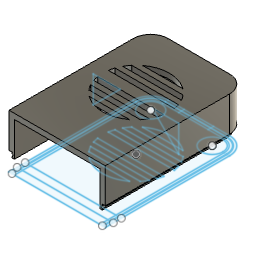
USB2CAN module enclosure v9 (Autodesk Fusion 360 design; units mm, degrees)
Autodesk Fusion 360 part; units mm, degrees
note: some values were not read from the file. Chosen so that the rebuilt part matches the saved one: which bodies a step acts on; which face or edge a step refers to.
sketch "PCB" plane through (0, 0, 0) normal (0, 0, 1) x (1, 0, 0)
  line L0 (-15.5, -25) -> (15.5, -25)
  line L1 (15.5, -25) -> (15.5, 21)
  line L2 (11.5, 25) -> (-11.5, 25)
  line L3 (-15.5, 21) -> (-15.5, -25)
  arc A0 (-11.5, 25) -> (-15.5, 21) centre (-11.5, 21) ccw
  arc A1 (15.5, 21) -> (11.5, 25) centre (11.5, 21) ccw
  circle A2 centre (-11.5, 21) radius 1.5
  circle A3 centre (11.5, 21) radius 1.5
  line L4 (-15.5, -24) -> (15.5, -24)
  circle A4 centre (0, 9) radius 1.75
  circle A5 centre (0, 9) radius 5
  dimension "d3" = 4
  dimension "d4" = 3
  dimension "d5" = 3
  dimension "d6" = -1
  dimension "d55" = 3.5
  dimension "d58" = 10
  constraint horizontal L0
  constraint perpendicular L0 L1
  constraint parallel L0 L2
  constraint parallel L1 L3
  constraint tangent L2 A0
  constraint tangent L3 A0
  constraint tangent L2 A1
  constraint tangent L1 A1
  constraint equal A0 A1
  constraint concentric A0 A2
  constraint concentric A1 A3
  constraint concentric A4 A5
  measures "d3" radius of A0
  measures "d4" diameter of A2
  measures "d5" diameter of A3
  measures "d55" diameter of A4
  measures "d58" diameter of A5
sketch "Base" plane through (0, 0, 0) normal (0, 0, 1) x (1, 0, 0)
  line L0 (11.5, 25.5) -> (-11.5, 25.5)
  arc A0 (-11.5, 25.5) -> (-16, 21) centre (-11.5, 21) ccw
  line L1 (-16, 21) -> (-16, -25.5)
  line L2 (-18, -25.5) -> (18, -25.5)
  line L3 (16, -25.5) -> (16, 21)
  arc A1 (16, 21) -> (11.5, 25.5) centre (11.5, 21) ccw
  line L4 (11.5, 27.5) -> (-11.5, 27.5)
  arc A2 (-11.5, 27.5) -> (-18, 21) centre (-11.5, 21) ccw
  line L5 (-18, 21) -> (-18, -25.5)
  line L6 (18, -25.5) -> (18, 21)
  arc A3 (18, 21) -> (11.5, 27.5) centre (11.5, 21) ccw
  line L7 (5.5, 25.5) -> (5.5, 27.5)
  line L8 (-5.5, 25.5) -> (-5.5, 27.5)
  line L9 (17.1, -25.5) -> (17.1, 21)
  arc A4 (17.1, 21) -> (11.5, 26.6) centre (11.5, 21) ccw
  line L10 (11.5, 26.6) -> (-11.5, 26.6)
  arc A5 (-11.5, 26.6) -> (-17.1, 21) centre (-11.5, 21) ccw
  line L11 (-17.1, 21) -> (-17.1, -25.5)
  line L12 (16.9, -25.5) -> (16.9, 21)
  arc A6 (16.9, 21) -> (11.5, 26.4) centre (11.5, 21) ccw
  line L13 (11.5, 26.4) -> (-11.5, 26.4)
  arc A7 (-11.5, 26.4) -> (-16.9, 21) centre (-11.5, 21) ccw
  line L14 (-16.9, 21) -> (-16.9, -25.5)
  dimension "d40" = 0.9
  constraint tangent A0 L1
  constraint tangent L0 A0
  constraint tangent L3 A1
  constraint tangent L0 A1
  constraint tangent L4 A2
  constraint tangent L6 A3
  constraint tangent A2 L5
  constraint tangent L4 A3
  constraint coincident L1.end L2
  constraint coincident L3.start L2
  constraint coincident L0 L8.start
  constraint coincident L0 L7.start
  constraint coincident L4 L7.end
  constraint coincident L4 L8.end
  constraint concentric A3 A4
  constraint concentric A2 A5
  constraint tangent A5 L11
  constraint tangent L10 A5
  constraint tangent A4 L10
  constraint tangent L9 A4
  constraint coincident L2 L11.end
  constraint coincident L2 L9.start
sketch "Supports" plane through (0, 0, 0) normal (0, 0, 1) x (1, 0, 0)
  line L0 (-16, -24) -> (16, -24)
  circle A0 centre (-11.5, 21) radius 1.25
  circle A1 centre (-11.5, 21) radius 2.5
  line L1 (-16, -25) -> (16, -25)
  circle A2 centre (11.5, 21) radius 2.5
  circle A3 centre (11.5, 21) radius 1.25
  line L2 (-16, -24) -> (-16, -25)
  line L3 (16, -24) -> (16, -25)
  dimension "d17" = 2.5
  dimension "d18" = 2.5
  dimension "d20" = 5
  dimension "d21" = 5
  dimension "d22" = 1
  constraint horizontal L1
  constraint perpendicular L1 L2
  constraint perpendicular L1 L3
  measures "d17" diameter of A0
  measures "d18" diameter of A3
  measures "d20" diameter of A1
  measures "d21" diameter of A2
  measures "d22" distance of L0 L1
extrude "Extrude1" add sketch "Base" along normal blind 1 contours L0 A0 L1 L2 L3 A1 makes body 1
extrude "Extrude2" add sketch "Base" along normal blind 5 contours L0 L2 L3 A1 L7 L12 A6 L13 | L0 A0 L1 L2 L8 L13 A7 L14 | L2 L7 L9 A4 L10 L12 A6 L13 | L2 L8 L10 A5 L11 L13 A7 L14 | L2 L4 L6 A3 L7 L9 A4 L10 | L2 L4 A2 L5 L8 L10 A5 L11 bodies 1
extrude "Extrude3" add sketch "Base" along normal blind 2 contours L0 L7 L8 L13 | L7 L8 L10 L13 | L4 L7 L8 L10 bodies 1
extrude "Extrude4" add sketch "Supports" along normal blind 3 bodies 1
extrude "Extrude5" cut sketch "Supports" along normal blind 5 contours A0 | A3 bodies 1
extrude "Extrude6" add sketch "Base" along normal blind 3 contours L0 L7 L8 L13 | L7 L8 L10 L13 | L4 L7 L8 L10 bodies 1
extrude "Extrude7" add sketch "Base" along normal blind 2 from surface at 5 contours L2 L4 L6 A3 L7 L9 A4 L10 | L2 L4 A2 L5 L8 L10 A5 L11 bodies 1
extrude "Extrude8" add sketch "Supports" along normal blind 5 contours A0 | A3 bodies 1
pipe "Pipe2" add diameter 0.75 path "Base" along L11 A5 L10 A4 L9 separate body makes body 2
move_body "Move2" bodies 2 to x (1, 0, 0) y (0, 1, 0) z (0, 0, 1) at (0, 0, 6)
split "Split1" by plane through (-5.5, 25.5, 0) normal (1, 0, 0) bodies 2 makes body 3 at (17.1151, -10, 5.6253)
split "Split2" by plane through (5.5, 25.5, 0) normal (-1, 0, 0) bodies 3 makes body 4 at (1.8333, 26.8481, 5.7188)
delete_body "RemoveBody1" bodies 4
combine "Combine1" operation add target body 1 tool bodies 2 3
extrude "Extrude9" cut sketch "PCB" along normal blind 2 contours A4 bodies 1
extrude "Extrude10" add sketch "PCB" against normal blind 1.5 contours L0 L1 L3 L4 | A2 | A3 | A5 bodies 1
sketch "Sketch4" plane through (0, 0, 0) normal (0, 0, 1) x (1, 0, 0)
  line L0 (11.5, 25.5) -> (-11.5, 25.5)
  line L1 (-16, 21) -> (-16, -25.5)
  line L2 (11.5, 27.5) -> (-11.5, 27.5)
  line L3 (11.5, 26.4) -> (-11.5, 26.4)
  line L4 (-5.5, 25.5) -> (-5.5, 27.5)
  line L5 (18, -25.5) -> (18, 21)
  arc A0 (18, 21) -> (11.5, 27.5) centre (11.5, 21) ccw
  arc A1 (16.9, 21) -> (11.5, 26.4) centre (11.5, 21) ccw
  line L6 (5.5, 25.5) -> (5.5, 27.5)
  arc A2 (-11.5, 25.5) -> (-16, 21) centre (-11.5, 21) ccw
  arc A3 (-11.5, 27.5) -> (-18, 21) centre (-11.5, 21) ccw
  line L7 (-18, 21) -> (-18, -25.5)
  arc A4 (-11.5, 26.6) -> (-17.1, 21) centre (-11.5, 21) ccw
  line L8 (17.1, -25.5) -> (17.1, 21)
  arc A5 (-11.5, 26.4) -> (-16.9, 21) centre (-11.5, 21) ccw
  line L9 (16, -25.5) -> (16, 21)
  line L10 (16.9, -25.5) -> (16.9, 21)
  line L11 (-17.1, 21) -> (-17.1, -25.5)
  arc A6 (17.1, 21) -> (11.5, 26.6) centre (11.5, 21) ccw
  line L12 (-16.9, 21) -> (-16.9, -25.5)
  line L13 (11.5, 26.6) -> (-11.5, 26.6)
  arc A7 (16, 21) -> (11.5, 25.5) centre (11.5, 21) ccw
  line L14 (-18, -25.5) -> (18, -25.5)
  circle A8 centre (-11.5, 21) radius 4
  circle A9 centre (11.5, 21) radius 4
  line L15 (12.339, 6) -> (-12.339, 6)
  line L16 (12.339, 2) -> (-12.339, 2)
  line L17 (11.8427, 0) -> (-11.8427, 0)
  line L18 (10.9659, -2) -> (-10.9659, -2)
  line L19 (9.6047, -4) -> (-9.6047, -4)
  line L20 (7.5, -6) -> (-7.5, -6)
  line L21 (11.8427, 8) -> (-11.8427, 8)
  line L22 (10.9659, 10) -> (-10.9659, 10)
  line L23 (9.6047, 12) -> (-9.6047, 12)
  line L24 (7.5, 14) -> (-7.5, 14)
  arc A10 (-7.5, -6) -> (7.5, -6) centre (0, 4) ccw
  arc A11 (7.5, 14) -> (-7.5, 14) centre (0, 4) ccw
  arc A12 (-9.6047, 12) -> (-10.9659, 10) centre (0, 4) ccw
  arc A13 (10.9659, 10) -> (9.6047, 12) centre (0, 4) ccw
  arc A14 (-11.8427, 8) -> (-12.339, 6) centre (0, 4) ccw
  arc A15 (12.339, 6) -> (11.8427, 8) centre (0, 4) ccw
  arc A16 (-12.339, 2) -> (-11.8427, 0) centre (0, 4) ccw
  arc A17 (-10.9659, -2) -> (-9.6047, -4) centre (0, 4) ccw
  arc A18 (9.6047, -4) -> (10.9659, -2) centre (0, 4) ccw
  arc A19 (11.8427, 0) -> (12.339, 2) centre (0, 4) ccw
  line L25 (-18, -22.5) -> (18, -22.5)
  line L26 (-18, -19.5) -> (18, -19.5)
  line L27 (-16, 4, 8) -> (-16, 4, 18)
  line L28 (16, 4, 8) -> (16, 4, 18)
  line L29 (-16, 4, 8) -> (-6, 4, 18)
  line L30 (6, 4, 18) -> (16, 4, 8)
  line L31 (-16, 4, 18) -> (-6, 4, 18)
  line L32 (6, 4, 18) -> (16, 4, 18)
  point P0 (0, 4)
  point P1 (0, 4)
  point P2 (0, 4)
  dimension "d61" = 0.9
  dimension "d62" = 0.9
  dimension "d63" = 0.9
  dimension "d64" = 0.9
  dimension "d65" = 8
  dimension "d66" = 8
  dimension "d69" = 25
  dimension "d96" = -3
  dimension "d97" = -6
  dimension "d103" = 10
  dimension "d104" = 10
  dimension "d105" = 10
  dimension "d106" = 10
  constraint coincident P2 P1
  constraint tangent L1 A2
  constraint tangent L0 A2
  constraint tangent L9 A7
  constraint tangent L0 A7
  constraint tangent L2 A3
  constraint tangent L5 A0
  constraint tangent A3 L7
  constraint tangent L2 A0
  constraint coincident L1.end L14
  constraint coincident L9.start L14
  constraint coincident L4.start L0
  constraint coincident L6.start L0
  constraint coincident L6.end L2
  constraint coincident L4.end L2
  constraint concentric A0 A6
  constraint concentric A3 A4
  constraint tangent A4 L11
  constraint tangent A4 L13
  constraint tangent A6 L13
  constraint tangent L8 A6
  constraint coincident L11.end L14
  constraint coincident L8.start L14
  constraint concentric A2 A8
  constraint concentric A0 A9
  constraint parallel L15 L21
  constraint concentric A10 A18
  constraint coincident L24.start A18
  constraint coincident L24.end A18
  constraint concentric A11 A18
  constraint concentric A11 A12
  constraint concentric A12 A14
  constraint concentric A13 A18
  constraint coincident L15.start A18
  constraint concentric A14 A16
  constraint concentric A15 A18
  constraint coincident L17.start A18
  constraint coincident L18.end A16
  constraint concentric A16 A17
  constraint concentric A18 A19
  measures "d62" distance of L5 L8
  measures "d63" distance of L2 L13
  measures "d64" distance of L7 L11
  measures "d65" diameter of A8
  measures "d66" diameter of A9
  measures "d69" diameter of A18
extrude "Extrude12" add sketch "Sketch4" against normal blind 1 from surface at 19 separate body contours L0 L1 A2 L9 A7 L26 | L0 L3 A1 L6 L9 L10 A7 L26 | L0 L3 L4 L6 | L0 L1 L3 L4 A2 A5 L12 L26 | L3 A1 L6 L8 L10 A6 L13 L26 | L3 L4 L6 L13 | L9 L10 L25 L26 | L1 L9 L25 L26 | L3 L4 A4 A5 L11 L12 L13 L26 | L2 L4 L6 L13 | L2 L5 A0 L6 L8 A6 L13 L26 | L9 L10 L14 L25 | L1 L9 L14 L25 | L1 L12 L25 L26 | L8 L10 L25 L26 | L2 L4 A3 L7 A4 L11 L13 L26 | L1 L12 L14 L25 | L8 L10 L14 L25 | L11 L12 L25 L26 | L5 L8 L25 L26 | L11 L12 L14 L25 | L5 L8 L14 L25 | L7 L11 L25 L26 | L7 L11 L14 L25 | A8 | A9 makes body 5
extrude "Extrude13" add sketch "Sketch4" along normal blind 4 from surface at 14 contours L0 L3 A1 L6 L9 L10 A7 L26 | L0 L3 L4 L6 | L0 L1 L3 L4 A2 A5 L12 L26 | L3 A1 L6 L8 L10 A6 L13 L26 | L3 L4 L6 L13 | L9 L10 L25 L26 | L3 L4 A4 A5 L11 L12 L13 L26 | L2 L4 L6 L13 | L2 L5 A0 L6 L8 A6 L13 L26 | L9 L10 L14 L25 | L1 L12 L25 L26 | L8 L10 L25 L26 | L2 L4 A3 L7 A4 L11 L13 L26 | L1 L12 L14 L25 | L8 L10 L14 L25 | L11 L12 L25 L26 | L5 L8 L25 L26 | L11 L12 L14 L25 | L5 L8 L14 L25 | L7 L11 L25 L26 | L7 L11 L14 L25 bodies 5
extrude "Extrude14" add sketch "Sketch4" along normal blind 3 from surface at 11 contours L0 L3 A1 L6 L9 L10 A7 L26 | L0 L1 L3 L4 A2 A5 L12 L26 | L3 A1 L6 L8 L10 A6 L13 L26 | L9 L10 L25 L26 | L3 L4 A4 A5 L11 L12 L13 L26 | L2 L5 A0 L6 L8 A6 L13 L26 | L9 L10 L14 L25 | L1 L12 L25 L26 | L8 L10 L25 L26 | L2 L4 A3 L7 A4 L11 L13 L26 | L1 L12 L14 L25 | L8 L10 L14 L25 | L11 L12 L25 L26 | L5 L8 L25 L26 | L11 L12 L14 L25 | L5 L8 L14 L25 | L7 L11 L25 L26 | L7 L11 L14 L25 bodies 5
move_body "Move3" bodies 5 to x (1, 0, 0) y (0, 1, 0) z (0, 0, 1) at (0, 0, -1)
move_face "OffsetFaces1" offset 3 1 faces at (16.6667, 5.5, 10) on bodies 5
move_face "OffsetFaces2" offset 3 1 faces at (-16.6667, -10, 10) on bodies 5
move_face "OffsetFaces3" offset 3 1 faces at (-1.8333, 26.1667, 13) on bodies 5
extrude "Extrude15" add sketch "Sketch4" against normal blind 1.9 from surface at 7 contours L0 L3 A1 L6 L9 L10 A7 L26 | L0 L1 L3 L4 A2 A5 L12 L26 | L9 L10 L25 L26 | L9 L10 L14 L25 | L1 L12 L25 L26 | L1 L12 L14 L25 bodies 5
pipe "Pipe3" add diameter 0.85 path "Sketch4" along L12 A5 L3 A1 L10 separate body makes body 6
move_body "Move4" bodies 6 to x (1, 0, 0) y (0, 1, 0) z (0, 0, 1) at (0, 0, 6)
combine "Combine2" operation cut target body 5 tool bodies 6
extrude "Extrude16" add sketch "Sketch4" against normal blind 12 from surface at 17 contours A8 | A9 bodies 5
move_face "OffsetFaces4" offset 1 1 faces at (-0.2977, -19.8227, 18) on bodies 5
split "Split3" by plane through (0, 0, 17) normal (0, 0, -1) bodies 5 makes body 7 at (15.495, 20.8006, 9) makes body 8 at (16, -10, 13.0333) makes body 9 at (-7.505, 20.8006, 9)
move_body "Move5" bodies 5 to x (1, 0, 0) y (0, 1, 0) z (0, 0, 1) at (0, 0, 1)
move_face "OffsetFaces5" offset 1 1 faces at (-17.3333, -10, 17) on bodies 8
move_face "OffsetFaces6" offset 1 2 faces at (11.2033, 22.2999, 17) (-13.4084, 19.5348, 17) on bodies 7 9
combine "Combine3" operation add target body 5 tool bodies 9 7 8
extrude "Extrude17" add sketch "Sketch4" along normal blind 1.5 separate body contours L1 L9 L25 L26 makes body 10
move_body "Move6" bodies 10 to x (1, 0, 0) y (0, 1, 0) z (0, 0, 1) at (0, 0, 16.5)
combine "Combine4" operation add target body 5 tool bodies 10
sketch "Sketch4 (curves on the plane with normal 0, 1, 0 at 4 mm)" plane through (0, 4, 0) normal (0, 1, 0) x (-1, 0, 0)
  line L0 (16, 8) -> (16, 18)
  line L1 (-16, 8) -> (-16, 18)
  line L2 (16, 8) -> (6, 18)
  line L3 (-6, 18) -> (-16, 8)
  line L4 (16, 18) -> (6, 18)
  line L5 (-6, 18) -> (-16, 18)
extrude "Extrude18" add sketch "Sketch4 (curves on the plane with normal 0, 1, 0 at 4 mm)" along normal mid plane 4 bodies 5
hidden bodies 1
equation "d104 = d103"
equation "d106 = d105"
